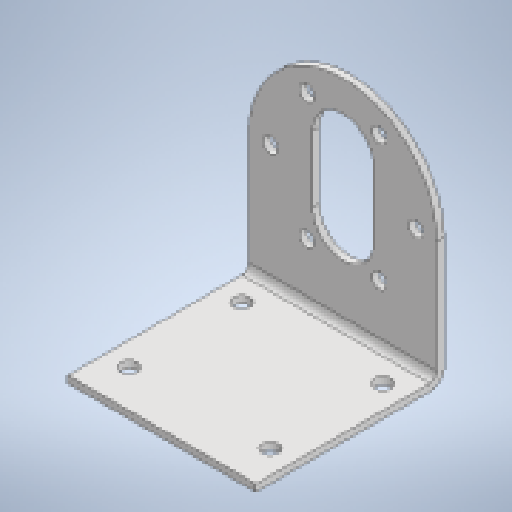
# Autodesk Inventor part: 电机支架
Saved by Autodesk Inventor 2025.1 (Build 291241000, 241)
## iProperties
Created: 2025-08-26
Part Number: 电机支架
Material: 常规
Document SubType Name: Modeling
Designer: Piw
Density: 1 g/cm^3
Appearance: 默认
Author: Piw
Autodesk Inventor part; units mm, degrees
ref_plane "YZ Plane" through (0, 0, 0) normal (1, 0, 0) x (0, 1, 0)
ref_plane "XZ Plane" through (0, 0, 0) normal (0, 1, 0) x (-1, 0, 0)
ref_plane "XY Plane" through (0, 0, 0) normal (0, 0, 1) x (1, 0, 0)
sketch "草图1" plane through (0, 0, 0) normal (0, 1, 0) x (-1, 0, 0)
  line L0 (-20, 20) -> (20, 20)
  line L1 (20, 20) -> (20, -20)
  line L2 (20, -20) -> (-20, -20)
  line L3 (-20, -20) -> (-20, 20)
  line L4 (-20, 20) -> (20, -20) construction
  line L5 (20, 20) -> (-20, -20) construction
  line L6 (0, 40.4687) -> (0, -51.5947)
  line L7 (-15, -12) -> (15, -12) construction
  line L8 (15, -12) -> (15, 12) construction
  line L9 (15, 12) -> (-15, 12) construction
  line L10 (-15, 12) -> (-15, -12) construction
  line L11 (-15, -12) -> (15, 12) construction
  line L12 (15, -12) -> (-15, 12) construction
  circle A0 centre (15, 12) radius 1.75
  circle A1 centre (15, -12) radius 1.75
  circle A2 centre (-15, -12) radius 1.75
  circle A3 centre (-15, 12) radius 1.75
  point P0 (0, 0)
  point P1 (0, 0)
  dimension "d0" = 40
  dimension "d1" = 40
  dimension "d2" = 8
  dimension "d3" = 24
  dimension "d4" = 30
  dimension "d5" = 3.5
  dimension "d6" = 3.5
  dimension "d7" = 3.5
  dimension "d8" = 3.5
  constraints: 26 end point, 4 centre point, 4 coincident, 4 midpoint, 4 parallel, 2 horizontal, 2 perpendicular, 2 vertical, 1 point on line
  measures "d0" distance of L1.end L2.end
  measures "d1" distance of L0.end L1.end
  measures "d2" distance between parallel lines of L0 L9
  measures "d3" distance between parallel lines of L7 L9
  measures "d4" distance between parallel lines of L10 L8
  measures "d5" diameter of A0
  measures "d6" diameter of A1
  measures "d7" diameter of A2
  measures "d8" diameter of A3
extrude "拉伸1" add sketch "草图1" along normal blind 1.5
sketch "草图3" plane through (20, 0, -20) normal (0, 0, -1) x (-1, 0, 0)
  line L0 (0, 0) -> (40, 0)
  line L1 (40, 0) -> (40, 27)
  line L2 (40, 47) -> (20, 47) construction
  line L3 (0, 27) -> (0, 0)
  line L4 (0, 0) -> (0, 1.5) projected
  line L5 (40, 0) -> (40, 1.5) projected
  arc A0 (40, 27) -> (0, 27) centre (20, 27) ccw
  line L6 (40, 27) -> (40, 47) construction
  line L7 (20, 20) -> (20, 34) construction
  line L8 (13.5, 20) -> (13.5, 34)
  line L9 (26.5, 34) -> (26.5, 20)
  arc A1 (13.5, 20) -> (26.5, 20) centre (20, 20) ccw
  arc A2 (26.5, 34) -> (13.5, 34) centre (20, 34) ccw
  circle A3 centre (20, 27) radius 15.5 construction
  circle A4 centre (4.5, 27) radius 1.6
  line L10 (20, 27) -> (4.5, 27) construction
  circle A5 centre (12.25, 13.5766) radius 1.6
  circle A6 centre (27.75, 13.5766) radius 1.6
  circle A7 centre (35.5, 27) radius 1.6
  circle A8 centre (27.75, 40.4234) radius 1.6
  circle A9 centre (12.25, 40.4234) radius 1.6
  point P0 (20, 0)
  dimension "d19" = 31
  dimension "d16" = 47
  dimension "d17" = 7
  dimension "d18" = 6.5
  dimension "d20" = 3.2
  dimension "d23" = 360
  constraints: 20 end point, 9 centre point, 8 tangent, 7 point on circle, 4 parallel, 3 collinear, 2 horizontal, 2 perpendicular, 1 coincident, 1 horizontal alignment, 1 midpoint, 1 vertical, 15 other
  measures "d16" distance of L0.end L2.start
  measures "d17" distance of A0.centre L7.end
  measures "d18" radius of A2
  measures "d20" diameter of A4
extrude "拉伸3" add sketch "草图3" against normal blind 1.5
fillet "圆角3" radius 3 1 edges at (0, 0, -20)
fillet "圆角4" radius 1.5 1 edges at (0, 1.5, -18.5)
